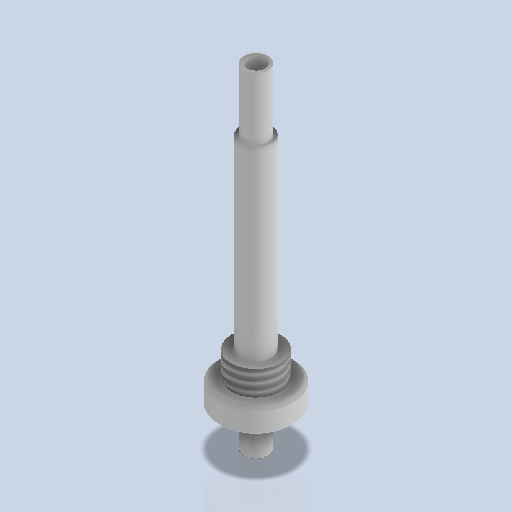
# Autodesk Inventor part: BRS
Saved by Autodesk Inventor 2024.2 (Build 282272000, 272)
## iProperties
Created: 2024-05-14
Part Number: BRS
Material: Generisch
Document SubType Name: Modeling
Designer: Fabri
Density: 1 g/cm^3
Appearance: Vorgabe
Author: Fabri
Autodesk Inventor part; units mm, degrees
ref_plane "YZ Plane" through (0, 0, 0) normal (1, 0, 0) x (0, 1, 0)
ref_plane "XZ Plane" through (0, 0, 0) normal (0, 1, 0) x (-1, 0, 0)
ref_plane "XY Plane" through (0, 0, 0) normal (0, 0, 1) x (1, 0, 0)
sketch "Skizze1" plane through (0, 0, 0) normal (0, 1, 0) x (-1, 0, 0)
  line L0 (0, 0) -> (0, -54)
  line L1 (0, 0) -> (2, 0)
  line L2 (2, 0) -> (2, -10)
  line L3 (2, -10) -> (2.5, -10)
  line L4 (2.5, -10) -> (2.5, -40)
  line L5 (2.5, -40) -> (4, -40)
  line L6 (4, -40) -> (4, -44)
  line L7 (4, -44) -> (6, -44)
  line L8 (6, -44) -> (6, -48)
  line L9 (6, -48) -> (2.5, -48)
  line L10 (2.5, -48) -> (2.5, -46)
  line L11 (2.5, -46) -> (2, -46)
  line L12 (2, -46) -> (2, -54)
  line L13 (2, -54) -> (0, -54)
  point P0 (0, -27)
  point P1 (4.25, -48)
  point P2 (3.25, -40)
  point P3 (1, -54)
  point P4 (1, 0)
  dimension "d0" = 54
  dimension "d1" = 36
  dimension "d2" = 4
  dimension "d3" = 4
  dimension "d4" = 4
  dimension "d5" = 12
  dimension "d6" = 5
  dimension "d7" = 8
  dimension "d8" = 8
  dimension "d11" = 10
  dimension "d12" = 6
  constraints: 29 end point, 10 perpendicular, 5 midpoint, 4 point on line, 1 horizontal, 1 vertical
  measures "d0" distance of L0.start L0.end
  measures "d1" distance of L11.end L2.end
  measures "d2" distance of L7.end L8.end
  measures "d3" distance from line of L7 L4.end
  measures "d4" diameter of L2 L0
  measures "d5" diameter of L8 L0
  measures "d6" diameter of L4 point (0, -27)
  measures "d7" diameter of L6 L0
  measures "d8" vertical distance of point (4.25, -48) point (3.25, -40)
  measures "d11" vertical distance of point (1, 0) L3.end
  measures "d12" distance from line of L12.end L9
revolve "Umdrehung1" add sketch "Skizze1" angle 360 about axis through (0, 0, 0) along (0, 0, -1)
thread "Gewinde1" size "M8x1.25" class "6g" standard "ISO Metric profile" length 18
chamfer "Fasen1" distance 0.5 angle 45 1 edges at (6, 0, -48)
chamfer "Fasen2" distance 0.5 angle 45 1 edges at (6, 0, -44)
sketch "Skizze2" plane through (0, 0, 0) normal (0, 0, 1) x (1, 0, 0)
  circle A0 centre (0, 0) radius 2 projected
  constraints: 1 coincident
hole "Bohrung1" at (0, 0, 0) direction (0, 0, -1) diameter 3 end through all
